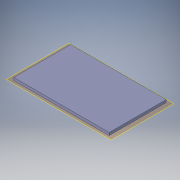
# Autodesk Inventor part: stamp5x3_empty
Saved by Autodesk Inventor 2019 (Build 230136000, 136)
## iProperties
Created: 2019-02-19
Part Number: stamp5x3_empty
Material: PET Plastic
Document SubType Name: Modeling
Designer: jmc
Density: 1.541 g/cm^3
Appearance: Slate Blue
Author: jmc
Autodesk Inventor part; units mm, degrees
ref_plane "YZ Plane" through (0, 0, 0) normal (1, 0, 0) x (0, 1, 0)
ref_plane "XZ Plane" through (0, 0, 0) normal (0, 1, 0) x (-1, 0, 0)
ref_plane "XY Plane" through (0, 0, 0) normal (0, 0, 1) x (1, 0, 0)
sketch "Sketch1" plane through (0, 0, 0) normal (0, 1, 0) x (-1, 0, 0)
  line L0 (24.925, 14.925) -> (-24.925, 14.925)
  line L1 (-24.925, 14.925) -> (-24.925, -14.925)
  line L2 (-24.925, -14.925) -> (24.925, -14.925)
  line L3 (24.925, 14.925) -> (-24.925, -14.925) construction
  line L4 (-24.925, 14.925) -> (24.925, -14.925) construction
  line L5 (24.925, -14.925) -> (24.925, 14.925)
  line L6 (24.925, 5) -> (24.925, 14.925)
  point P0 (0, 0)
  dimension "d0" = 49.85
  dimension "d1" = 29.85
  constraints: 14 end point, 3 parallel, 2 midpoint, 1 horizontal, 1 perpendicular
  measures "d0" distance of L2.end L1.end
  measures "d1" distance of L1.end L0.end
extrude "Extrusion1" add sketch "Sketch1" along normal blind 1.4
sketch "Sketch2" plane through (0, 0, 0) normal (0, -1, 0) x (1, 0, 0)
  point P0 (0, 0)
sketch "Sketch3" plane through (-24.925, 0, -14.925) normal (-1, 0, 0) x (0, 0, 1)
  point P0 (14.925, 0)
ref_plane "Work Plane1" through (0, 0, 0) normal (0, 1, 0) x (-1, 0, 0)
sketch "Sketch5" plane through (0, 0, 0) normal (0, 1, 0) x (-1, 0, 0)
  line L0 (-24.925, 14.925) -> (24.925, 14.925) projected
  line L1 (24.925, -14.925) -> (-24.925, -14.925) projected
  line L2 (24.925, 14.925) -> (24.925, -14.925) projected
  line L3 (-19.3821, 7.7039) -> (19.3821, 7.7039) construction
  line L4 (19.3821, 7.7039) -> (19.3821, -7.7039) construction
  line L5 (19.3821, -7.7039) -> (-19.3821, -7.7039) construction
  line L6 (-19.3821, -7.7039) -> (-19.3821, 7.7039) construction
  line L7 (-24.925, -14.925) -> (-24.925, 14.925) projected
  point P0 (0, 0)
  dimension "d13" = 29.85
  dimension "d14" = 49.85
  dimension "d16" = 38.7641
  dimension "d17" = 15.4078
  dimension "d18" = 7.2211
  dimension "d22" = 5.5429
  constraints: 2 other
  measures "d13" distance between parallel lines of L1 L0
  measures "d14" distance of L0.start L0.end
  measures "d16" distance of L3.start L3.end
  measures "d17" distance of L3.end L4.end
  measures "d18" distance between parallel lines of L0 L3
  measures "d22" distance between parallel lines of L7 L6
sketch "Sketch6" plane through (0, 0, 0) normal (0, -1, 0) x (1, 0, 0)
  line L0 (-24.925, 14.925) -> (-24.925, -14.925) projected
  line L1 (24.925, 14.925) -> (-24.925, 14.925) projected
  line L2 (24.925, -14.925) -> (24.925, 14.925) projected
  line L3 (-24.925, -14.925) -> (24.925, -14.925) projected
  line L4 (-22.925, 10.925) -> (-22.925, -10.925)
  line L5 (-20.925, -12.925) -> (20.925, -12.925)
  line L6 (22.925, -10.925) -> (22.925, 10.925)
  line L7 (20.925, 12.925) -> (-20.925, 12.925)
  arc A0 (-20.925, 12.925) -> (-22.925, 10.925) centre (-20.925, 10.925) ccw
  arc A1 (-22.925, -10.925) -> (-20.925, -12.925) centre (-20.925, -10.925) ccw
  arc A2 (20.925, -12.925) -> (22.925, -10.925) centre (20.925, -10.925) ccw
  arc A3 (22.925, 10.925) -> (20.925, 12.925) centre (20.925, 10.925) ccw
  line L8 (-20.925, 12.525) -> (20.925, 12.525)
  arc A4 (22.525, 10.925) -> (20.925, 12.525) centre (20.925, 10.925) ccw
  line L9 (22.525, 10.925) -> (22.525, -10.925)
  arc A5 (20.925, -12.525) -> (22.525, -10.925) centre (20.925, -10.925) ccw
  line L10 (20.925, -12.525) -> (-20.925, -12.525)
  arc A6 (-22.525, -10.925) -> (-20.925, -12.525) centre (-20.925, -10.925) ccw
  line L11 (-22.525, -10.925) -> (-22.525, 10.925)
  arc A7 (-20.925, 12.525) -> (-22.525, 10.925) centre (-20.925, 10.925) ccw
  point P0 (0, 0)
  dimension "d23" = 2
  dimension "d24" = 2
  dimension "d25" = 0.4
  constraints: 16 end point, 16 point on circle, 8 centre point, 8 tangent, 3 equal radius, 10 other
  measures "d23" distance between parallel lines of L1 L7
  measures "d24" radius of A0
  measures "d25" distance between parallel lines of L7 L8
equation "\"d18\" = 0.5 * d13 - 0.5 * d17"
equation "\"d22\" = 0.5 * d14 - 0.5 * d16"
body "Solid1"
